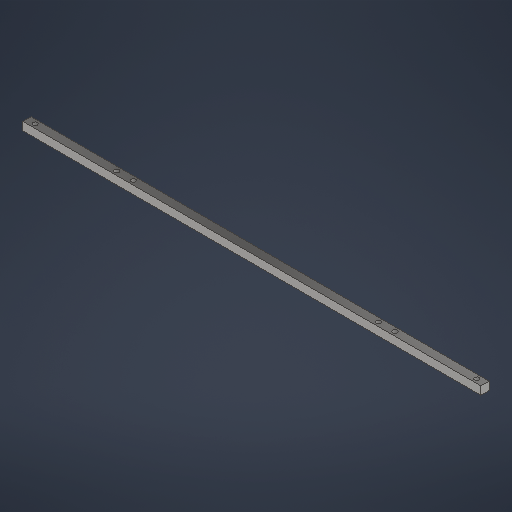
# Autodesk Inventor part: Chassis Cross Brace
Saved by Autodesk Inventor 2026.2 (Build 302298000, 298)
## iProperties
Created: 2025-11-12
Part Number: Chassis Cross Brace
Material: Steel
Document SubType Name: Modeling
Designer: T. TYLER
Density: 7.85 g/cm^3
Appearance: Steel - Polished
Engr Approved By: E. BISSELL
Engineer: E. BISSELL
Mass: 111.56 g
Surface Area: 92.1532 cm^2
Volume: 14.2114 cm^3
Author: T. TYLER
Title: Chassis Cross Brace
Autodesk Inventor part; units mm, degrees
ref_plane "YZ Plane" through (0, 0, 0) normal (1, 0, 0) x (0, 1, 0)
ref_plane "XZ Plane" through (0, 0, 0) normal (0, 1, 0) x (-1, 0, 0)
ref_plane "XY Plane" through (0, 0, 0) normal (0, 0, 1) x (1, 0, 0)
sketch "Sketch1" plane through (0, 0, 0) normal (1, 0, 0) x (0, 1, 0)
  line L0 (0, 0) -> (6.35, 0)
  line L1 (6.35, 0) -> (6.35, -6.35)
  line L2 (6.35, -6.35) -> (0, -6.35)
  line L3 (0, -6.35) -> (0, 0)
  dimension "d0" = 6.35
  dimension "d1" = 6.35
  constraints: 8 end point, 2 parallel, 1 horizontal, 1 perpendicular
  measures "d0" distance of L1.end L2.end
  measures "d1" distance of L0.end L1.end
extrude "Extrusion1" add sketch "Sketch1" along normal blind 355.6
sketch "Sketch2" plane through (0, 6.35, 0) normal (0, 1, 0) x (1, 0, 0)
  circle A0 centre (6.35, 3.175) radius 1.7859
  line L0 (0, 6.35) -> (0, 0) projected
  line L1 (0, 0) -> (355.6, 0) projected
  circle A1 centre (349.25, 3.175) radius 1.7859
  line L2 (355.6, 6.35) -> (355.6, 0) projected
  circle A2 centre (82.55, 3.175) radius 1.7859
  circle A3 centre (273.05, 3.175) radius 1.7859
  circle A4 centre (285.75, 3.175) radius 1.8021
  circle A5 centre (69.85, 3.175) radius 1.786
  dimension "d4" = 3.5719
  dimension "d5" = 6.35
  dimension "d6" = 3.175
  dimension "d7" = 3.5719
  dimension "d8" = 6.35
  dimension "d9" = 3.175
  dimension "d16" = 3.5719
  dimension "d17" = 3.175
  dimension "d18" = 76.2
  dimension "d19" = 3.5719
  dimension "d20" = 3.175
  dimension "d21" = 76.2
  dimension "d26" = 12.7
  dimension "d27" = 12.7
  constraints: 6 centre point
  measures "d4" diameter of A0
  measures "d5" distance from line of L0 A0.centre
  measures "d6" distance from line of L1 A0.centre
  measures "d7" diameter of A1
  measures "d8" distance from line of L2 A1.centre
  measures "d9" distance from line of L1 A1.centre
  measures "d16" diameter of A2
  measures "d17" distance from line of L1 A2.centre
  measures "d18" distance of A0.centre A2.centre
  measures "d19" diameter of A3
  measures "d20" distance from line of L1 A3.centre
  measures "d21" distance of A1.centre A3.centre
  measures "d26" distance of A3.centre A4.centre
  measures "d27" distance of A2.centre A5.centre
extrude "Extrusion2" cut sketch "Sketch2" against normal through all
thread "Thread1" size "8-32 UNC" class "2B" standard "ANSI Unified Screw Threads" full length
thread "Thread2" size "8-32 UNC" class "2B" standard "ANSI Unified Screw Threads" full length
thread "Thread3" size "8-32 UNC" class "2B" standard "ANSI Unified Screw Threads" full length
thread "Thread4" size "8-32 UNC" class "2B" standard "ANSI Unified Screw Threads" full length
thread "Thread5" size "8-32 UNC" class "2B" standard "ANSI Unified Screw Threads" full length
thread "Thread6" size "8-32 UNC" class "2B" standard "ANSI Unified Screw Threads" full length
body "Solid1"
